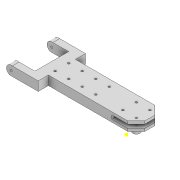
# Autodesk Inventor part: RobotBaseMotorExt
Saved by Autodesk Inventor 2022 (Build 260153000, 153)
## iProperties
Created: 2022-10-20
Part Number: RobotBaseMotorExt
Material: Generic
Document SubType Name: Modeling
Designer: MVeszpremi
Density: 1 g/cm^3
Appearance: Default
Author: MVeszpremi
Autodesk Inventor part; units mm, degrees
sketch "Sketch1" plane through (0, 0, 0) normal (0, 1, 0) x (-1, 0, 0)
  line L0 (0, 0) -> (145, 0)
  line L1 (145, 0) -> (145, -70)
  line L2 (145, -70) -> (0, -70)
  line L3 (0, -70) -> (0, 0)
  line L4 (10, -25) -> (30, -25)
  line L5 (30, -25) -> (30, -45)
  line L6 (30, -45) -> (10, -45)
  line L7 (10, -45) -> (10, -25)
  circle A0 centre (10, -25) radius 1.5
  circle A1 centre (30, -45) radius 1.5
  circle A2 centre (30, -25) radius 1.5
  circle A3 centre (10, -45) radius 1.5
  line L8 (145, 0) -> (130, 0)
  line L9 (130, 0) -> (130, -70)
  line L10 (130, -70) -> (145, -70)
  line L11 (145, -70) -> (145, 0)
  line L12 (130, -15) -> (0, -15)
  line L13 (0, -15) -> (0, -55)
  line L14 (0, -55) -> (130, -55)
  line L15 (130, -55) -> (130, -15)
  line L16 (36, -15) -> (36, -55)
  point P0 (130, 0)
  point P1 (0, -15)
  dimension "d0" = 145
  dimension "d1" = 70
  dimension "d2" = 20
  dimension "d3" = 20
  dimension "d4" = 25
  dimension "d5" = 10
  dimension "d6" = 3
  dimension "d7" = 3
  dimension "d8" = 3
  dimension "d9" = 3
  dimension "d18" = 15
  dimension "d19" = 15
  dimension "d23" = 36
  dimension "d66" = 15
  constraints: 34 end point, 8 parallel, 5 perpendicular, 5 point on line, 4 centre point, 4 coincident, 4 horizontal
  measures "d0" distance of L1.end L2.end
  measures "d1" distance of L0.end L1.end
  measures "d2" distance of L4.start L4.end
  measures "d3" distance of L4.end L5.end
  measures "d4" distance between parallel lines of L0 L4
  measures "d5" distance between parallel lines of L3 L7
  measures "d6" diameter of A2
  measures "d7" diameter of A1
  measures "d8" diameter of A3
  measures "d9" diameter of A0
  measures "d18" distance between parallel lines of L0 L12
  measures "d19" distance between parallel lines of L2 L14
  measures "d23" distance between parallel lines of L13 L16
  measures "d66" distance between parallel lines of L1 L9
extrude "Extrusion1" add sketch "Sketch1" along normal blind 4 contours L0 L1 L2 L9 | L12 L16 L14 L3 | L9 L14 L16 L12 | L4 A2 L5 A1 L6 A3 L7 A0
extrude "Extrusion2" add sketch "Sketch1" against normal blind 5.5 contours L0 L1 L2 L9 | L9 L14 L16 L12
ref_plane "Work Plane1" through (0, -2.75, 0) normal (0, -1, 0) x (1, 0, 0)
mirror "Mirror1" about plane through (0, -2.75, 0) normal (0, -1, 0) of "Extrusion1"
chamfer "Chamfer1" distance 12.5 angle 45 4 edges at (0, 2, -15) (0, -7.5, -15) (0, -7.5, -55) (0, 2, -55)
ref_plane "Work Plane2" through (-152.5, -8.5, -20) normal (0, 0, -1) x (-1, 0, 0)
sketch "Sketch5" plane through (-130, -9.5, -55) normal (0, -1, 0) x (1, 0, 0)
  circle A0 centre (100, 30) radius 1.5 projected
  line L0 (100, 33.4641) -> (103, 31.7321)
  line L1 (103, 31.7321) -> (103, 28.2679)
  line L2 (103, 28.2679) -> (100, 26.5359)
  line L3 (100, 26.5359) -> (97, 28.2679)
  line L4 (97, 28.2679) -> (97, 31.7321)
  line L5 (97, 31.7321) -> (100, 33.4641)
  circle A1 centre (120, 30) radius 1.5 projected
  line L6 (120, 33.4641) -> (123, 31.7321)
  line L7 (123, 31.7321) -> (123, 28.2679)
  line L8 (123, 28.2679) -> (120, 26.5359)
  line L9 (120, 26.5359) -> (117, 28.2679)
  line L10 (117, 28.2679) -> (117, 31.7321)
  line L11 (117, 31.7321) -> (120, 33.4641)
  circle A2 centre (120, 10) radius 1.5 projected
  line L12 (120, 13.4641) -> (123, 11.7321)
  line L13 (123, 11.7321) -> (123, 8.2679)
  line L14 (123, 8.2679) -> (120, 6.5359)
  line L15 (120, 6.5359) -> (117, 8.2679)
  line L16 (117, 8.2679) -> (117, 11.7321)
  line L17 (117, 11.7321) -> (120, 13.4641)
  circle A3 centre (100, 10) radius 1.5 projected
  line L18 (100, 13.4641) -> (103, 11.7321)
  line L19 (103, 11.7321) -> (103, 8.2679)
  line L20 (103, 8.2679) -> (100, 6.5359)
  line L21 (100, 6.5359) -> (97, 8.2679)
  line L22 (97, 8.2679) -> (97, 11.7321)
  line L23 (97, 11.7321) -> (100, 13.4641)
  circle A4 centre (100, 30) radius 5.25
  circle A5 centre (120, 30) radius 5.25
  circle A6 centre (120, 10) radius 5.25
  circle A7 centre (100, 10) radius 5.25
  point P0 (130, 55)
  dimension "d44" = 6
  dimension "d45" = 6
  dimension "d46" = 6
  dimension "d47" = 6
  dimension "d48" = 10.5
  dimension "d49" = 10.5
  dimension "d50" = 10.5
  dimension "d51" = 10.5
  constraints: 48 end point, 8 coincident, 4 centre point, 52 other
  measures "d44" distance between parallel lines of L1 L4
  measures "d45" distance between parallel lines of L7 L10
  measures "d46" distance between parallel lines of L13 L16
  measures "d47" distance between parallel lines of L19 L22
  measures "d48" diameter of A4
  measures "d49" diameter of A5
  measures "d50" diameter of A7
  measures "d51" diameter of A6
extrude "Extrusion5" add sketch "Sketch5" along normal blind 3.5 contours A4 | A5 | A6 | A7
sketch "Sketch6" plane through (-130, -9.5, -55) normal (0, -1, 0) x (1, 0, 0)
  circle A0 centre (0, 10) radius 1.5
  line L0 (117.5, 0) -> (0, 0) projected
  line L1 (0, 0) -> (0, -15) projected
  circle A1 centre (20, 10) radius 1.5
  circle A2 centre (40, 10) radius 1.5
  circle A3 centre (60, 10) radius 1.5
  point P0 (130, 55)
  point P1 (0, -5)
  dimension "d54" = 3
  dimension "d55" = 10
  dimension "d56" = 0
  dimension "d59" = 20
  constraints: 4 centre point, 1 horizontal, 6 other
  measures "d54" diameter of A0
  measures "d55" distance from line of L0 A0.centre
  measures "d56" distance from line of L1 A0.centre
  measures "d59" distance of A0.centre A1.centre
extrude "Extrusion6" cut sketch "Sketch6" against normal blind 33.25
ref_plane "Work Plane3" through (-130, -9.5, -35) normal (0, 0, -1) x (-1, 0, 0)
mirror "Mirror2" about plane through (-130, -9.5, -35) normal (0, 0, -1) of "Extrusion6"
sketch "Sketch7" plane through (-145, 4, 0) normal (0, 0, 1) x (1, 0, 0)
  point P0 (145, -4)
sketch "Sketch8" plane through (-145, 4, 0) normal (0, 0, 1) x (1, 0, 0)
  line L0 (0, 0) -> (15, 0) projected
  line L1 (15, 0) -> (0, 0) projected
  circle A0 centre (-25, -6.7937) radius 1.5
  circle A1 centre (-25, -6.7937) radius 7
  line L2 (0, -13.5) -> (0, 0) projected
  line L3 (0, -13.5) -> (0, 0) projected
  line L4 (-50, -13.5875) -> (0, -13.5875)
  line L5 (0, -13.5875) -> (0, 0)
  line L6 (0, 0) -> (-50, 0)
  line L7 (-50, 0) -> (-50, -13.5875)
  line L8 (-50, -13.5875) -> (0, 0) construction
  line L9 (0, -13.5875) -> (-50, 0) construction
  point P0 (145, -4)
  point P1 (-10, -1.851)
  point P2 (-10, -11.649)
  point P3 (-26.6868, -13.5875)
  point P4 (-26.6868, 0)
  point P5 (-23.3132, 0)
  point P6 (-23.3132, -13.5875)
  dimension "d72" = 3
  dimension "d73" = 14
  dimension "d74" = 25
  constraints: 12 end point, 2 centre point, 2 midpoint, 2 parallel, 1 coincident, 1 horizontal, 1 perpendicular
  measures "d72" diameter of A0
  measures "d73" diameter of A1
  measures "d74" distance from line of L2 A0.centre
extrude "Extrusion7" add sketch "Sketch8" against normal blind 10 contours A1 L4 L6 | A1 L6 L2 L5 L4 | L6 A1 | A1 L4
ref_plane "Work Plane4" through (-130, -9.5, -35) normal (0, 0, 1) x (1, 0, 0)
mirror "Mirror3" about plane through (-130, -9.5, -35) normal (0, 0, 1) of "Extrusion7"
body "Solid1"
